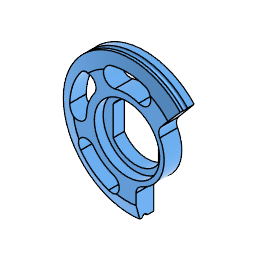
Driver Wheel_ (Autodesk Fusion 360 design; units mm, degrees)
Autodesk Fusion 360 part; units mm, degrees
sketch "Sketch1" plane through (0, 0, 0) normal (1, 0, 0) x (0, 1, 0)
  line L0 (2.25, 0) -> (9, 0)
  line L1 (9, 0) -> (9, 13)
  line L2 (9, 13) -> (10, 13)
  line L3 (8, 13.0018) -> (8, 30.0018)
  line L4 (0.1376, 24.0019) -> (0.043, 7.5003)
  line L5 (2.25, 0) -> (0.043, 7.5003)
  line L6 (1.772, 30.0018) -> (0.1376, 24.0019)
  arc A0 (3, 30.0018) -> (5, 30.0018) centre (4, 30.0018) ccw
  line L7 (8, 30.0018) -> (5, 30.0018)
  line L8 (3, 30.0018) -> (1.772, 30.0018)
  line L9 (0.043, 7.5003) -> (0, 0)
  line L10 (0, 0) -> (2.25, 0)
  line L11 (2.25, 0) -> (9, 0)
  line L12 (9, 13) -> (9, 0)
  line L13 (9, 13) -> (8, 13.0018)
  point P0 (0.172, 30.0018)
  dimension "d1" = 9
  dimension "d2" = 13
  dimension "d3" = 17
  dimension "d4" = 1
  dimension "d5" = 2.25
  dimension "d6" = 7.5005
  dimension "d7" = 1.6
  dimension "d8" = 6
  dimension "d9" = 1
  dimension "d10" = 3
  constraint coincident L9.end L10.start
  constraint horizontal L0
  constraint perpendicular L0 L1
  constraint perpendicular L1 L2
  constraint perpendicular L2 L3
  constraint perpendicular L3 L7
  constraint coincident L9.end L0
  constraint coincident L9.end L4
  constraint coincident P0 L7
  constraint coincident P0 L4
  constraint coincident A0.start L7
  constraint collinear L7 L8
  constraint coincident A0.centre L7
  measures "d1" distance of L9.end L0.end
  measures "d2" distance of L0.end L1.end
  measures "d3" distance of L3.start L3.end
  measures "d4" distance of L1.end L3.start
  measures "d5" distance of L9.end L0.start
  measures "d6" distance of L9.end L4.end
  measures "d7" distance of P0 L6.start
  measures "d8" distance of P0 L4.start
  measures "d9" radius of A0
  measures "d10" distance of L3.end A0.end
revolve "Revolve1" add sketch "Sketch1" angle 360 about axis through (0, 2.25, 0) along (0, 1, 0)
sketch "Sketch2" plane through (0, 0, 0) normal (0, 1, 0) x (1, 0, 0)
  arc A0 (-5.3869, -16.5801) -> (5.1945, -16.313) centre (-0.5171, 0.2287) ccw
  arc A1 (-5.3869, -16.5801) -> (-7.6131, -24.2641) centre (-6.5, -20.4221) ccw
  arc A2 (-7.6131, -24.2641) -> (7.8055, -23.8749) centre (-0.5171, 0.2287) ccw
  arc A3 (7.8055, -23.8749) -> (5.1945, -16.313) centre (6.5, -20.094) ccw
  arc A4 (-6.5, -20.4221) -> (6.5, -20.094) centre (-0.5171, 0.2287) ccw construction
  arc A5 (-26.0101, -0.3689) -> (-21.0025, -14.9569) centre (-0.5171, 0.2287) ccw
  arc A6 (-21.0025, -14.9569) -> (-14.5757, -10.1928) centre (-17.7891, -12.5748) ccw
  arc A7 (-18.0123, -0.1814) -> (-14.5757, -10.1928) centre (-0.5171, 0.2287) ccw
  arc A8 (-18.0123, -0.1814) -> (-26.0101, -0.3689) centre (-22.0112, -0.2752) ccw
  arc A9 (-8.7529, 24.3621) -> (-21.1599, 15.1995) centre (-0.5171, 0.2287) ccw
  arc A10 (-21.1599, 15.1995) -> (-14.6837, 10.5028) centre (-17.9218, 12.8512) ccw
  arc A11 (-6.1692, 16.7908) -> (-14.6837, 10.5028) centre (-0.5171, 0.2287) ccw
  arc A12 (-6.1692, 16.7908) -> (-8.7529, 24.3621) centre (-7.461, 20.5765) ccw
  line L0 (0, 0) -> (0, -45.0987) construction
  line L1 (0, 0) -> (49.3466, 0) construction
  circle A13 centre (0, 0) radius 16.5
  line L2 (22, -20.3988) -> (15.0673, -12.1367)
  arc A14 (14.5936, -7.6991) -> (15.0673, -12.1367) centre (18.1315, -9.5655) ccw
  line L3 (4, 29.734) -> (4, 18.8746)
  arc A15 (4, 18.8746) -> (6.439, 15.1917) centre (8, 18.8746) ccw
  circle A16 centre (0, 0) radius 30.0018
  dimension "d12" = 4
  dimension "d13" = 25.5
  dimension "d14" = 6.5
  dimension "d15" = 6.5
  dimension "d17" = -145
  dimension "d18" = 33
  dimension "d19" = 140
  dimension "d20" = 4
  dimension "d21" = 4
  dimension "d22" = 4
  dimension "d23" = 22
  constraint tangent A0 A1
  constraint tangent A1 A2
  constraint tangent A2 A3
  constraint tangent A0 A3
  constraint coincident L0.start L1.start
  constraint vertical L0
  constraint perpendicular L0 L1
  constraint coincident A13 A14.start
  constraint tangent L2 A14
  constraint tangent A13 A14
  constraint vertical L3
  constraint coincident A13 A15.end
  constraint tangent L3 A15
  constraint tangent A13 A15
  constraint coincident L3.start A16
  constraint coincident L2.start A16
  measures "d12" radius of A1
  measures "d13" radius of A2
  measures "d14" horizontal distance of L0.start A1.centre
  measures "d15" horizontal distance of L0.start A3.centre
  measures "d18" diameter of A13
  measures "d19" angle of L2 L3
  measures "d20" radius of A15
  measures "d21" radius of A14
  measures "d22" distance of L0.start L3
  measures "d23" distance of L0 L2.start
extrude "Extrude1" cut sketch "Sketch2" along normal up to surface (8 mm away) contours A0 A1 A2 A3 | A5 A6 A7 A8 | A9 A10 A11 A12 | A13 L2 A14 L3 A15 A16 picked at (8.2829, 20.1154)
sketch "Sketch3" plane through (0, 8, 0) normal (0, 1, 0) x (-1, 0, 0)
  line L0 (-4, -18.8746) -> (-4, -29.734)
  arc A0 (-4, -29.734) -> (-22, 20.3988) centre (0, 0) ccw
  line L1 (-22, 20.3988) -> (-15.0673, 12.1367)
  arc A1 (-14.5936, 7.6991) -> (-15.0673, 12.1367) centre (-18.1315, 9.5655) ccw
  arc A2 (-14.5936, 7.6991) -> (-6.439, -15.1917) centre (0, 0) ccw
  arc A3 (-4, -18.8746) -> (-6.439, -15.1917) centre (-8, -18.8746) ccw
  arc A4 (26.0101, 0.3689) -> (21.0025, 14.9569) centre (0.5171, -0.2287) ccw
  arc A5 (18.0123, 0.1814) -> (26.0101, 0.3689) centre (22.0112, 0.2752) ccw
  arc A6 (18.0123, 0.1814) -> (14.5757, 10.1928) centre (0.5171, -0.2287) ccw
  arc A7 (21.0025, 14.9569) -> (14.5757, 10.1928) centre (17.7891, 12.5748) ccw
  arc A8 (8.7529, -24.3621) -> (21.1599, -15.1995) centre (0.5171, -0.2287) ccw
  arc A9 (6.1692, -16.7908) -> (8.7529, -24.3621) centre (7.461, -20.5765) ccw
  arc A10 (6.1692, -16.7908) -> (14.6837, -10.5028) centre (0.5171, -0.2287) ccw
  arc A11 (21.1599, -15.1995) -> (14.6837, -10.5028) centre (17.9218, -12.8512) ccw
  arc A12 (7.6131, 24.2641) -> (-7.8055, 23.8749) centre (0.5171, -0.2287) ccw
  arc A13 (5.3869, 16.5801) -> (7.6131, 24.2641) centre (6.5, 20.4221) ccw
  arc A14 (5.3869, 16.5801) -> (-5.1945, 16.313) centre (0.5171, -0.2287) ccw
  arc A15 (-7.8055, 23.8749) -> (-5.1945, 16.313) centre (-6.5, 20.094) ccw
  circle A16 centre (0, 0) radius 13.0018
  line L2 (10.05, 6.5572) -> (10.05, -6.5572)
  line L3 (-10.05, 6.5572) -> (-10.05, -6.5572)
  line L4 (0, 0) -> (0, 20.9906) construction
  arc A17 (10.05, 6.5572) -> (-10.05, 6.5572) centre (0, 0) ccw
  arc A18 (-10.05, -6.5572) -> (10.05, -6.5572) centre (0, 0) ccw
  dimension "d26" = 24
  dimension "d27" = 20.1
  constraint coincident A0.centre A2.centre
  constraint vertical L2
  constraint coincident L3.end A17
  constraint parallel L2 L3
  constraint symmetric L2 L3 L4
  constraint concentric A17 A18
  measures "d26" diameter of A17
  measures "d27" distance of L2 L3
extrude "Extrude2" cut sketch "Sketch3" along normal blind -76 and the other way blind -16 contours L2 L3 A17 A18
sketch "Sketch6" plane through (0, 0, 0) normal (0, 1, 0) x (1, 0, 0)
  circle A0 centre (0, 0) radius 14.5
  line L0 (10.05, -6.5573) -> (10.05, 6.5573)
  line L1 (0, 0) -> (0, -5.2001) construction
  line L2 (-10.05, -6.5573) -> (-10.05, 6.5573)
  arc A1 (10.05, -6.5573) -> (10.05, 6.5573) centre (0, 0) ccw
  arc A2 (-10.05, 6.5573) -> (-10.05, -6.5573) centre (0, 0) ccw
  dimension "d36" = 29
  dimension "d37" = 24
  constraint coincident A0.centre L1.start
  constraint vertical L0
  constraint parallel L0 L1
  constraint symmetric L0.start L1 L2.start
  constraint symmetric L0.end L1 L2.end
  constraint concentric A1 A2
  measures "d36" diameter of A0
  measures "d37" diameter of A1
extrude "Extrude4" cut sketch "Sketch6" along normal blind 4 contours A0 | L0 A1 | L2 A2
extrude "Extrude3" [suppressed]
